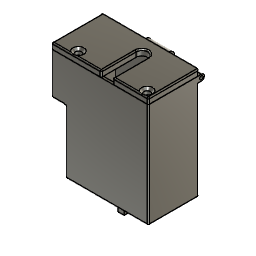
housing final project v8 (Autodesk Fusion 360 design; units mm, degrees)
Autodesk Fusion 360 part; units mm, degrees
note: some values were not read from the file. Set by a fixed rule: which face or edge a step refers to.
sketch "Sketch1" plane through (0, 0, 0) normal (0, 0, 1) x (1, 0, 0)
  line L0 (0, 0) -> (66.04, 0)
  line L1 (66.04, 0) -> (66.04, 38.1)
  line L2 (66.04, 38.1) -> (0, 38.1)
  line L3 (0, 38.1) -> (0, 0)
  line L4 (25.57, 28.525) -> (27.77, 28.525)
  line L5 (27.77, 28.525) -> (27.77, 19.825)
  line L6 (27.77, 19.825) -> (25.57, 19.825)
  line L7 (25.57, 19.825) -> (25.57, 28.525)
  line L8 (38.27, 27.675) -> (40.47, 27.675)
  line L9 (40.47, 27.675) -> (40.47, 20.675)
  line L10 (40.47, 20.675) -> (38.27, 20.675)
  line L11 (38.27, 20.675) -> (38.27, 27.675)
  line L12 (30.32, 12.275) -> (35.72, 12.275) construction
  line L13 (35.72, 12.275) -> (35.72, 9.575)
  line L14 (35.72, 9.575) -> (30.32, 9.575)
  line L15 (30.32, 9.575) -> (30.32, 12.275)
  line L16 (26.67, 28.525) -> (26.67, 19.825) construction
  line L17 (39.37, 27.675) -> (39.37, 20.675) construction
  arc A0 (35.72, 12.275) -> (30.32, 12.275) centre (33.02, 12.275) ccw
  line L18 (40.47, 24.175) -> (38.27, 24.175) construction
  line L19 (25.57, 24.175) -> (27.77, 24.175) construction
  dimension "d1" = 66.04
  dimension "d2" = 38.1
  dimension "d3" = 8.7
  dimension "d4" = 2.2
  dimension "d5" = 7
  dimension "d6" = 2.2
  dimension "d7" = 12.7
  dimension "d8" = 5.4
  dimension "d9" = 5.4
  dimension "d10" = 2.7
  dimension "d11" = 2.7
  dimension "d12" = 11.9
  dimension "d13" = 6.35
  dimension "d14" = 33.02
  dimension "d15" = 9.575
  constraint horizontal L0
  constraint vertical L1
  constraint horizontal L2
  constraint vertical L3
  constraint coincident L0.start L3.end
  constraint horizontal L4
  constraint vertical L5
  constraint horizontal L6
  constraint vertical L7
  constraint horizontal L8
  constraint vertical L9
  constraint horizontal L10
  constraint vertical L11
  constraint horizontal L12
  constraint vertical L13
  constraint horizontal L14
  constraint vertical L15
  constraint midpoint L4 L16.start
  constraint midpoint L6 L16.end
  constraint midpoint L8 L17.start
  constraint midpoint L10 L17.end
  constraint tangent L13 A0
  constraint midpoint L9 L18.start
  constraint midpoint L11 L18.end
  constraint midpoint L7 L19.start
  constraint midpoint L5 L19.end
  constraint collinear L18 L19
  measures "d1" distance of L1.end L2.end
  measures "d2" distance of L0.end L1.end
  measures "d3" distance of L4 L6
  measures "d4" distance of L4.start L4.end
  measures "d5" distance of L8.start L10.end
  measures "d6" distance of L8.start L8.end
  measures "d7" distance of L16 L17
  measures "d8" distance of L13.end L14.end
  measures "d9" diameter of A0
  measures "d10" distance of L14 A0.centre
  measures "d11" distance of L12.end L13.end
  measures "d12" distance of L12.end L18
  measures "d13" distance of L16 A0.centre
  measures "d14" distance of L1 A0.centre
  measures "d15" distance of L2 L4
extrude "Extrude1" add sketch "Sketch1" against normal blind 40.64 contours L0 L1 L2 L3 | L4 L5 L6 L7 | L8 L9 L10 L11 | L13 L14 L15 A0 makes body 1
extrude "Extrude2" cut sketch "Sketch1" against normal blind 15 contours L4 L5 L6 L7 | L8 L9 L10 L11 | L13 L14 L15 A0 bodies 1
extrude "Extrude3" add sketch "Sketch1" against normal blind 15 from surface at -40.64 contours L4 L5 L6 L7 | L8 L9 L10 L11 | L13 L14 L15 A0 bodies 1
sketch "Sketch3" plane through (25.57, 0, 0) normal (-1, 0, 0) x (0, -1, 0)
  line L0 (-19.825, -40.64) -> (-28.525, -40.64)
  circle A0 centre (-24.175, -50.64) radius 2
  line L1 (-24.175, -55.14) -> (-24.175, -40.64) construction
  line L2 (-28.525, -40.64) -> (-28.525, -55.64)
  line L3 (-28.525, -55.64) -> (-19.825, -55.64)
  line L4 (-19.825, -55.64) -> (-19.825, -40.64)
  dimension "d43" = 4
  constraint midpoint L0 L1.end
  constraint coincident A0.centre L1
  measures "d43" diameter of A0
sketch "Sketch2" plane through (66.04, 0, 0) normal (1, 0, 0) x (0, 1, 0)
  line L0 (35.1, -3) -> (3, -37.64) construction
  line L1 (35.1, -37.64) -> (3, -3) construction
  line L2 (25.55, -26.82) -> (12.55, -26.82)
  line L3 (12.55, -26.82) -> (12.55, -13.82)
  line L4 (12.55, -13.82) -> (25.55, -13.82)
  line L5 (25.55, -13.82) -> (25.55, -26.82)
  line L6 (25.55, -26.82) -> (12.55, -13.82) construction
  line L7 (12.55, -26.82) -> (25.55, -13.82) construction
  circle A0 centre (24.05, -15.32) radius 1.5
  line L8 (25.55, -20.32) -> (12.55, -20.32) construction
  line L9 (19.05, -13.82) -> (19.05, -26.82) construction
  circle A1 centre (24.05, -25.32) radius 1.5
  circle A2 centre (14.05, -15.32) radius 1.5
  circle A3 centre (14.05, -25.32) radius 1.5
  line L10 (38.1, 0) -> (0, 0)
  line L11 (0, 0) -> (0, -40.64)
  line L12 (0, -40.64) -> (38.1, -40.64)
  line L13 (38.1, -40.64) -> (38.1, 0)
  point P0 (19.05, -20.32)
  dimension "d27" = 13
  dimension "d28" = 13
  dimension "d29" = 3
  constraint horizontal L2
  constraint perpendicular L2 L3
  constraint parallel L2 L4
  constraint parallel L3 L5
  constraint coincident L6 P0
  constraint coincident L7 P0
  constraint tangent L5 A0
  constraint tangent L4 A0
  constraint midpoint L5 L8.start
  constraint midpoint L3 L8.end
  constraint midpoint L4 L9.start
  constraint midpoint L2 L9.end
  constraint symmetric A0 L8 A1
  constraint symmetric A0 L9 A2
  constraint symmetric L9 A1 A3
  constraint midpoint L1 P0
  measures "d27" distance of L2.start L2.end
  measures "d28" distance of L2.start L4.end
  measures "d29" diameter of A0
extrude "Extrude6" cut sketch "Sketch3" against normal up to surface (14.9 mm away) contours A0 bodies 1
extrude "Extrude5" add sketch "Sketch2" against normal blind 1 from surface at -66.04 contours L2 L3 L4 L5 A0 A1 A2 A3 | A1 | A3 | A0 | A2 bodies 1
extrude "Extrude4" add sketch "Sketch2" along normal blind 1 contours L2 L3 L4 L5 A0 A1 A2 A3 | A1 | A3 | A0 | A2 bodies 1
sketch "Sketch5" plane through (0, 0, -40.64) normal (0, 0, -1) x (1, 0, 0)
  line L0 (30.32, -12.275) -> (30.32, -9.575)
  line L1 (30.32, -9.575) -> (35.72, -9.575)
  line L2 (35.72, -9.575) -> (35.72, -12.275)
  arc A0 (30.32, -12.275) -> (35.72, -12.275) centre (33.02, -12.275) ccw
  line L3 (40.47, -27.675) -> (38.27, -27.675)
  line L4 (38.27, -27.675) -> (38.27, -20.675)
  line L5 (38.27, -20.675) -> (40.47, -20.675)
  line L6 (40.47, -20.675) -> (40.47, -27.675)
  line L7 (27.77, -28.525) -> (25.57, -28.525)
  line L8 (25.57, -28.525) -> (25.57, -19.825)
  line L9 (25.57, -19.825) -> (27.77, -19.825)
  line L10 (27.77, -19.825) -> (27.77, -28.525)
  line L11 (0, 0) -> (0, -38.1)
  line L12 (0, -38.1) -> (66.04, -38.1)
  line L13 (66.04, -38.1) -> (66.04, 0)
  line L14 (66.04, 0) -> (0, 0)
  line L15 (-0.5, -38.6) -> (66.54, -38.6)
  line L16 (66.54, -38.6) -> (66.54, 0.5)
  line L17 (66.54, 0.5) -> (-0.5, 0.5)
  line L18 (-0.5, 0.5) -> (-0.5, -38.6)
  line L19 (-2.5, 2.5) -> (-2.5, -40.6)
  line L20 (-2.5, -40.6) -> (68.54, -40.6)
  line L21 (68.54, -40.6) -> (68.54, 2.5)
  line L22 (68.54, 2.5) -> (-2.5, 2.5)
  dimension "d47" = 0.5
  dimension "d48" = 0.5
  dimension "d49" = 0.5
  dimension "d50" = 0.5
  dimension "d51" = 2
  constraint horizontal L15
  constraint vertical L16
  constraint horizontal L17
  constraint vertical L18
  measures "d47" distance of L13 L16
  measures "d48" distance of L11 L18
  measures "d49" distance of L12 L15
  measures "d50" distance of L14 L17
fillet "Fillet2" radius 1.5 4 edges at (26.67, 28.525, -55.64) (26.67, 19.825, -55.64) (39.37, 20.675, -55.64) (39.37, 27.675, -55.64) on bodies 1
fillet "Fillet3" radius 0.5 10 edges at (38.27, 20.675, -47.39) (38.27, 21.1143, -55.2007) (38.27, 24.175, -55.64) (38.27, 27.2357, -55.2007) (38.27, 27.675, -47.39) (40.47, 27.675, -47.39) (40.47, 27.2357, -55.2007) (40.47, 24.175, -55.64) (40.47, 21.1143, -55.2007) (40.47, 20.675, -47.39) on bodies 1
fillet "Fillet4" radius 0.5 10 edges at (27.77, 28.525, -47.39) (27.77, 28.0857, -55.2007) (27.77, 24.175, -55.64) (27.77, 20.2643, -55.2007) (27.77, 19.825, -47.39) (25.57, 19.825, -47.39) (25.57, 20.2643, -55.2007) (25.57, 24.175, -55.64) (25.57, 28.0857, -55.2007) (25.57, 28.525, -47.39) on bodies 1
fillet "Fillet5" radius 0.5 4 edges at (30.32, 10.925, -55.64) (33.02, 14.975, -55.64) (35.72, 10.925, -55.64) (33.02, 9.575, -55.64) on bodies 1
fillet "Fillet1" radius 3 12 edges at (0, 19.05, 0) (33.02, 38.1, 0) (66.04, 19.05, 0) (33.02, 0, 0) (0, 38.1, -20.32) (0, 0, -20.32) (0, 19.05, -40.64) (33.02, 0, -40.64) (66.04, 0, -20.32) (66.04, 19.05, -40.64) (66.04, 38.1, -20.32) (33.02, 38.1, -40.64) on bodies 1
chamfer "Chamfer1" distance 0.5 angle 45 12 edges at (26.67, 28.525, 0) (25.57, 24.175, 0) (27.77, 24.175, 0) (26.67, 19.825, 0) (39.37, 27.675, 0) (38.27, 24.175, 0) (40.47, 24.175, 0) (39.37, 20.675, 0) (33.02, 14.975, 0) (35.72, 10.925, 0) (30.32, 10.925, 0) (33.02, 9.575, 0) on bodies 1
extrude "Extrude7" add sketch "Sketch5" against normal blind 90 separate body contours L19 L20 L21 L22 makes body 2
sketch "Sketch6" plane through (-2.5, 0, 0) normal (-1, 0, 0) x (0, -1, 0)
  line L0 (-40.6, -40.64) -> (2.5, -40.64)
  line L1 (2.5, -40.64) -> (2.5, 49.36)
  line L2 (2.5, 49.36) -> (-40.6, 49.36)
  line L3 (-40.6, 49.36) -> (-40.6, -40.64)
  line L4 (-40.6, 0.36) -> (2.5, 0.36)
  line L5 (-40.6, 2.36) -> (2.5, 2.36)
  line L6 (-7.5, 2.36) -> (-7.5, 0.36)
  line L7 (-30.6, 2.36) -> (-30.6, 0.36)
  dimension "d54" = 41
  dimension "d55" = 2
  dimension "d56" = 10
  dimension "d57" = 10
  constraint coincident L3 L4.start
  constraint coincident L1 L4.end
  constraint perpendicular L1 L4
  constraint coincident L3 L5.start
  constraint coincident L1 L5.end
  constraint perpendicular L1 L5
  constraint coincident L5 L6.start
  constraint coincident L4 L6.end
  constraint perpendicular L4 L6
  constraint coincident L5 L7.start
  constraint coincident L4 L7.end
  constraint perpendicular L4 L7
  measures "d54" distance of L0 L4
  measures "d55" distance of L4 L5
  measures "d56" distance of L1 L6
  measures "d57" distance of L3 L7
extrude "Extrude8" add sketch "Sketch6" against normal blind 10 from surface at -2 contours L3 L4 L5 L7 | L1 L4 L5 L6 | L4 L5 L6 L7 bodies 2
extrude "Extrude9" add sketch "Sketch6" along normal blind 10 from surface at -69.04 contours L3 L4 L5 L7 | L1 L4 L5 L6 | L4 L5 L6 L7 bodies 2
chamfer "Chamfer2" distance 10 angle 45 2 edges at (-0.5, 19.05, 2.36) (66.54, 19.05, 2.36) on bodies 2
sketch "Sketch8" plane through (68.54, 0, 0) normal (1, 0, 0) x (0, 1, 0)
  line L0 (-2.5, -40.64) -> (40.6, -40.64)
  line L1 (40.6, -40.64) -> (40.6, 49.36)
  line L2 (40.6, 49.36) -> (-2.5, 49.36)
  line L3 (-2.5, 49.36) -> (-2.5, -40.64)
  line L4 (40.6, 49.36) -> (43.1, 49.36)
  line L5 (43.1, 49.36) -> (43.1, 44.36)
  line L6 (43.1, 44.36) -> (40.6, 44.36)
  line L7 (40.6, 44.36) -> (40.6, 49.36)
  circle A0 centre (43.1, 46.86) radius 2.5
  circle A1 centre (43.1, 46.86) radius 1.5
  line L8 (-2.5, 49.36) -> (7.5, 49.36)
  line L9 (7.5, 49.36) -> (7.5, 39.36)
  line L10 (7.5, 39.36) -> (-2.5, 39.36)
  line L11 (-2.5, 39.36) -> (-2.5, 49.36)
  line L12 (-0.5, 39.36) -> (-0.5, 49.36)
  dimension "d65" = 5
  dimension "d66" = 2.5
  dimension "d67" = 5
  dimension "d73" = 3
  dimension "d76" = 10
  dimension "d77" = 10
  dimension "d78" = 2
  constraint horizontal L4
  constraint vertical L5
  constraint horizontal L6
  constraint vertical L7
  constraint coincident L1.end L2.start
  constraint midpoint L5 A0.centre
  constraint concentric A0 A1
  constraint horizontal L8
  constraint vertical L9
  constraint horizontal L10
  constraint vertical L11
  constraint coincident L2.end L3.start
  constraint coincident L10 L12.start
  constraint coincident L8 L12.end
  constraint perpendicular L8 L12
  measures "d65" distance of L4.end L5.end
  measures "d66" distance of L1.end L4.end
  measures "d67" diameter of A0
  measures "d73" diameter of A1
  measures "d76" distance of L9.end L10.end
  measures "d77" distance of L8.end L9.end
  measures "d78" distance of L11 L12
extrude "Extrude10" add sketch "Sketch8" against normal blind 25 contours L1 L6 L7 A0 | L1 L4 L7 A0 | L5 A0 A1 | L5 A0 A1 | L5 A1 | L5 A1 bodies 2
extrude "Extrude11" add sketch "Sketch8" along normal blind 25 from surface at -71.04 contours L1 L6 L7 A0 | L1 L4 L7 A0 | L5 A0 A1 | L5 A0 A1 | L5 A1 | L5 A1 bodies 2
extrude "Extrude12" cut sketch "Sketch8" against normal up to surface (71.04 mm away) contours L5 A1 | L5 A1 bodies 2
extrude "Extrude13" add sketch "Sketch8" against normal blind 10 from surface at -2 contours L2 L8 L9 L10 L12 bodies 2
extrude "Extrude14" add sketch "Sketch8" along normal blind 10 from surface at -69.04 contours L2 L8 L9 L10 L12 bodies 2
sketch "Sketch10" plane through (-2.5, 0, 0) normal (-1, 0, 0) x (0, -1, 0)
  circle A0 centre (-43.1, 46.86) radius 1.5
  line L0 (-40.6, -40.64) -> (2.5, -40.64)
  line L1 (2.5, -40.64) -> (2.5, 49.36)
  line L2 (2.5, 49.36) -> (-43.1, 49.36)
  arc A1 (-43.1, 49.36) -> (-43.1, 44.36) centre (-43.1, 46.86) ccw
  line L3 (-43.1, 44.36) -> (-40.6, 44.36)
  line L4 (-40.6, 44.36) -> (-40.6, -40.64)
  line L5 (2.5, 54.46) -> (-40.6, 54.46)
  line L6 (-40.6, 54.46) -> (-40.6, 49.46)
  line L7 (-40.6, 49.46) -> (2.5, 49.46)
  line L8 (2.5, 49.46) -> (2.5, 54.46)
  line L9 (2.5, 39.36) -> (2.5, 49.36)
  circle A2 centre (-43.1, 46.86) radius 2.5
  dimension "d88" = 0.1
  dimension "d89" = 5
  constraint horizontal L5
  constraint vertical L6
  constraint horizontal L7
  constraint vertical L8
  constraint collinear L8 L9
  constraint collinear L4 L6
  measures "d88" distance of L2 L7
  measures "d89" distance of L5.start L7.end
extrude "Extrude16" add sketch "Sketch10" against normal up to surface (71.04 mm away) separate body contours L5 L6 L7 L8 makes body 3
sketch "Sketch12" plane through (0, 40.6, 0) normal (0, 1, 0) x (-1, 0, 0)
  line L0 (-68.54, 54.46) -> (-68.54, 49.46)
  line L1 (-68.54, 49.46) -> (2.5, 49.46)
  line L2 (2.5, 49.46) -> (2.5, 54.46)
  line L3 (2.5, 54.46) -> (-68.54, 54.46)
  line L4 (-33.02, 54.46) -> (-33.02, 49.46) construction
  line L5 (-23.02, 54.46) -> (-23.02, 49.46)
  line L6 (-43.02, 54.46) -> (-43.02, 49.46)
  dimension "d92" = 10
  constraint midpoint L3 L4.start
  constraint midpoint L1 L4.end
  constraint coincident L3 L5.start
  constraint coincident L1 L5.end
  constraint perpendicular L1 L5
  constraint symmetric L4 L5.start L6.start
  constraint symmetric L4 L5.end L6.end
  measures "d92" distance of L4 L5
extrude "Extrude17" add sketch "Sketch12" along normal blind 5 contours L1 L3 L5 L6 bodies 3
sketch "Sketch14" plane through (23.02, 0, 0) normal (-1, 0, 0) x (0, -1, 0)
  line L0 (-40.6, 49.46) -> (-40.6, 54.46)
  line L1 (-40.6, 54.46) -> (-45.6, 54.46)
  line L2 (-45.6, 54.46) -> (-45.6, 49.46)
  line L3 (-45.6, 49.46) -> (-40.6, 49.46)
  line L4 (-45.6, 49.46) -> (-40.6, 49.46)
  line L5 (-40.6, 49.46) -> (-40.6, 44.36)
  line L6 (-40.6, 44.36) -> (-45.6, 44.36)
  line L7 (-45.6, 44.36) -> (-45.6, 49.46)
  line L8 (-40.6, 49.36) -> (-45.6, 49.36)
  line L9 (-45.6, 49.36) -> (-40.6, 44.36) construction
  line L10 (-40.6, 49.36) -> (-45.6, 44.36) construction
  circle A0 centre (-43.1, 46.86) radius 2.5
  circle A1 centre (-43.1, 46.86) radius 1.5
  dimension "d96" = 5.1
  dimension "d97" = 5
  dimension "d98" = 0.1
  dimension "d99" = 5
  dimension "d100" = 3
  constraint horizontal L4
  constraint vertical L5
  constraint horizontal L6
  constraint vertical L7
  constraint coincident L2.end L3.start
  constraint coincident L5 L8.start
  constraint coincident L7 L8.end
  constraint perpendicular L7 L8
  constraint midpoint L10 A0.centre
  constraint concentric A0 A1
  measures "d96" distance of L2.end L6.end
  measures "d97" distance of L5.end L6.end
  measures "d98" distance of L4 L8
  measures "d99" diameter of A0
  measures "d100" diameter of A1
sketch "Sketch9" plane through (0, 0, 49.36) normal (0, 0, 1) x (-1, 0, 0)
  line L0 (0.5, -7.5) -> (0.5, -38.6)
  line L1 (0.5, -38.6) -> (-66.54, -38.6)
  line L2 (-66.54, -38.6) -> (-66.54, -7.5)
  line L3 (-66.54, -7.5) -> (-56.54, -7.5)
  line L4 (-56.54, -7.5) -> (-56.54, 0.5)
  line L5 (-56.54, 0.5) -> (-9.5, 0.5)
  line L6 (-9.5, 0.5) -> (-9.5, -7.5)
  line L7 (-9.5, -7.5) -> (0.5, -7.5)
  line L8 (2.5, 2.5) -> (-68.54, 2.5)
  line L9 (-68.54, 2.5) -> (-68.54, -43.1)
  line L10 (-68.54, -43.1) -> (-43.54, -43.1)
  line L11 (-43.54, -43.1) -> (-43.54, -40.6)
  line L12 (-43.54, -40.6) -> (-22.5, -40.6)
  line L13 (-22.5, -40.6) -> (-22.5, -43.1)
  line L14 (-22.5, -43.1) -> (2.5, -43.1)
  line L15 (2.5, -43.1) -> (2.5, 2.5)
  line L16 (-9.5, -7.5) -> (2.5, 2.5) construction
  line L17 (0.5, -7.5) -> (2.5, -7.5) construction
  line L18 (-9.5, 0.5) -> (-9.5, 2.5) construction
  line L19 (-9.5, 2.5) -> (2.5, -7.5) construction
  circle A0 centre (-3.5, -2.5) radius 2.7
  line L20 (-33.02, 2.5) -> (-33.02, 0.5) construction
  circle A1 centre (-62.54, -2.5) radius 2.7
  dimension "d85" = 5.4
  constraint coincident L6.end L7.start
  constraint coincident L8.start L15.end
  constraint coincident L0.start L7.end
  constraint coincident L15 L17.end
  constraint perpendicular L15 L17
  constraint coincident L5.end L6.start
  constraint coincident L8 L18.end
  constraint perpendicular L8 L18
  constraint midpoint L16 A0.centre
  constraint midpoint L8 L20.start
  constraint midpoint L5 L20.end
  constraint symmetric A0 L20 A1
  measures "d85" diameter of A0
extrude "Extrude15" cut sketch "Sketch9" against normal up to surface (10 mm away) contours A0 | A1 bodies 2
extrude "Extrude18" add sketch "Sketch14" against normal up to surface (20 mm away) contours L3 L4 L5 L7 L8 | L5 L8 A0 | L7 L8 A0 | A0 bodies 3
extrude "Extrude19" cut sketch "Sketch9" along normal up to surface (5.1 mm away) contours A0 | A1 bodies 3
sketch "Sketch15" plane through (0, 0, 54.46) normal (0, 0, 1) x (-1, 0, 0)
  circle A0 centre (-3.5, -2.5) radius 2.7
  circle A1 centre (-62.54, -2.5) radius 2.7
  line L0 (-68.54, 2.5) -> (-68.54, -40.6)
  line L1 (-68.54, -40.6) -> (-43.02, -40.6)
  line L2 (-43.02, -40.6) -> (-43.02, -45.6)
  line L3 (-43.02, -45.6) -> (-23.02, -45.6)
  line L4 (-23.02, -45.6) -> (-23.02, -40.6)
  line L5 (-23.02, -40.6) -> (2.5, -40.6)
  line L6 (2.5, -40.6) -> (2.5, 2.5)
  line L7 (2.5, 2.5) -> (-68.54, 2.5)
  line L8 (-33.02, -45.6) -> (-33.02, 2.5) construction
  line L9 (-38.02, -27.5) -> (-28.02, -27.5)
  line L10 (-28.02, -27.5) -> (-28.02, 2.5)
  line L11 (-28.02, 2.5) -> (-38.02, 2.5)
  line L12 (-38.02, 2.5) -> (-38.02, -27.5)
  line L13 (-38.02, -27.5) -> (-28.02, 2.5) construction
  line L14 (-28.02, -27.5) -> (-38.02, 2.5) construction
  circle A2 centre (-33.02, -27.5) radius 5
  point P0 (-33.02, -12.5)
  dimension "d107" = 30
  dimension "d108" = 10
  dimension "d109" = 10
  constraint midpoint L3 L8.start
  constraint midpoint L7 L8.end
  constraint horizontal L9
  constraint perpendicular L9 L10
  constraint parallel L9 L11
  constraint parallel L10 L12
  constraint coincident L13 P0
  constraint coincident L14 P0
  constraint coincident L8 P0
  constraint collinear L7 L11
  constraint midpoint L9 A2.centre
  measures "d107" distance of L9.start L11.end
  measures "d108" distance of L9.start L9.end
  measures "d109" diameter of A2
extrude "Extrude20" cut sketch "Sketch15" against normal up to surface (5 mm away) contours L7 L10 L11 L12 A2 | L9 A2 | L9 A2 bodies 3
fillet "Fillet6" radius 5 1 edges at (33.02, 45.6, 54.46) on bodies 3
chamfer "Chamfer3" distance 2 angle 45 2 edges at (6.0173, 1.5236, 54.46) (65.0573, 1.5236, 54.46) on bodies 3
sketch "Sketch19" plane through (-2.5, 0, 0) normal (-1, 0, 0) x (0, -1, 0)
  line L0 (-40.6, -40.64) -> (2.5, -40.64)
  line L1 (2.5, 49.36) -> (-43.1, 49.36)
  arc A0 (-43.1, 49.36) -> (-43.1, 44.36) centre (-43.1, 46.86) ccw
  line L2 (-43.1, 44.36) -> (-40.6, 44.36)
  circle A1 centre (-43.1, 46.86) radius 1.5
  line L3 (-2.3867, 49.36) -> (-2.3867, 15.36)
  line L4 (-2.3867, 15.36) -> (-36.3867, 15.36)
  line L5 (-36.3867, 15.36) -> (-36.3867, 49.36)
  line L6 (-19.05, -40.64) -> (-19.05, 49.36) construction
  line L7 (2.5, -40.64) -> (2.5, 49.36)
  line L8 (-40.6, 44.36) -> (-40.6, -40.64)
  line L9 (-40.6, 13.36) -> (2.5, 13.36)
  line L10 (-40.6, 44.36) -> (-40.6, 49.36)
  dimension "d140" = 34
  dimension "d141" = 34
  dimension "d156" = 2
  constraint vertical L3
  constraint horizontal L4
  constraint vertical L5
  constraint midpoint L0 L6.start
  constraint coincident L1 L6.end
  constraint perpendicular L1 L6
  constraint coincident L1 L3.start
  constraint coincident L8 L9.start
  constraint coincident L7 L9.end
  constraint perpendicular L7 L9
  constraint coincident L2.end L8.start
  constraint coincident L1 L10.end
  constraint perpendicular L1 L10
  measures "d140" distance of L5.end L3.start
  measures "d141" distance of L5.end L4.end
  measures "d156" distance of L4 L9
extrude "Extrude22" add sketch "Sketch19" along normal blind 10 contours L1 L3 L4 L5 L7 L8 L9 L10 bodies 2
extrude "Extrude23" add sketch "Sketch19" along normal blind 2 from surface at 10 contours L1 L3 L4 L5 L7 L8 L9 L10 | L1 L3 L4 L5 bodies 2
extrude "Extrude24" add 1 faces at (-2.5, 26.2333, 51.1267) along direction (-1, 0, 0) blind 12 on bodies 3 bodies 3
fillet "Fillet8" radius 1 3 edges at (68.54, 40.6, 1.86) (-2.5, 40.6, -13.64) (-2.5, 40.6, 46.86) on bodies 2
fillet "Fillet8" radius 1 11 edges at (-14.5, -2.5, 31.36) (-8.5, -2.5, 13.36) (-14.5, 19.05, 13.36) (-14.5, 40.6, 31.36) (-8.5, 40.6, 13.36) (-2.5, 19.05, 13.36) (-2.5, -2.5, -13.64) (-2.5, 19.05, -40.64) (33.02, -2.5, -40.64) (33.02, 40.6, -40.64) (68.54, 19.05, -40.64) on bodies 2
fillet "Fillet8" radius 1 1 edges at (68.54, -2.5, 4.36) on bodies 2
fillet "Fillet9" radius 1 8 edges at (68.54, 40.6, 51.96) (68.54, 19.05, 54.46) (68.54, -2.5, 51.96) (53.28, -2.5, 54.46) (28.02, 12.5, 54.46) (33.02, 32.5, 54.46) (38.02, 12.5, 54.46) (38.02, -2.5, 51.96) on bodies 3
fillet "Fillet9" radius 1 5 edges at (6.76, -2.5, 54.46) (-14.5, 19.05, 54.46) (-14.5, 40.6, 51.96) (-14.5, -2.5, 51.96) (28.02, -2.5, 51.96) on bodies 3
sketch "Sketch21" plane through (0, 40.6, 0) normal (0, 1, 0) x (-1, 0, 0)
  line L0 (3.5, 49.36) -> (3.5, 44.36)
  line L1 (3.5, 44.36) -> (-22.5, 44.36)
  line L2 (-22.5, 44.36) -> (-22.5, 49.36)
  line L3 (-22.5, 49.36) -> (-43.54, 49.36)
  line L4 (-43.54, 49.36) -> (-43.54, 44.36)
  line L5 (-43.54, 44.36) -> (-67.54, 44.36)
  line L6 (-67.54, 44.36) -> (-67.54, -39.64)
  line L7 (-67.54, -39.64) -> (1.5, -39.64)
  line L8 (1.5, -39.64) -> (1.5, 12.36)
  arc A0 (3.5, 14.36) -> (1.5, 12.36) centre (3.5, 12.36) ccw
  line L9 (3.5, 14.36) -> (13.5, 14.36)
  line L10 (13.5, 14.36) -> (13.5, 49.36)
  line L11 (13.5, 49.36) -> (3.5, 49.36)
  line L12 (-58.02, 5.36) -> (-8.02, 5.36)
  line L13 (-8.02, 5.36) -> (-8.02, -19.64)
  line L14 (-8.02, -19.64) -> (-58.02, -19.64)
  line L15 (-58.02, -19.64) -> (-58.02, 5.36)
  line L16 (-33.02, -39.64) -> (-33.02, 50.36) construction
  line L17 (-49.0719, 15.4014) -> (-17.0719, 15.4014) construction
  line L18 (-17.0719, 15.4014) -> (-17.0719, 29.4014) construction
  line L19 (-17.0719, 29.4014) -> (-49.0719, 29.4014) construction
  line L20 (-49.0719, 29.4014) -> (-49.0719, 15.4014) construction
  dimension "d163" = 25
  dimension "d164" = 50
  dimension "d165" = 20
  dimension "d166" = 8
  text T0 "Lacime" font "Arial" height 8 italic align centre top in box 32 x 14 at (-49.0719, 15.4014) x (1, 0) y (0, 1) spacing 1 kerned
  constraint horizontal L12
  constraint vertical L13
  constraint horizontal L14
  constraint vertical L15
  constraint midpoint L7 L16.start
  constraint perpendicular L7 L16
  constraint midpoint L12 L16
  measures "d163" distance of L12.end L13.end
  measures "d164" distance of L12.start L12.end
  measures "d165" distance of L7 L14
extrude "Extrude25" cut sketch "Sketch21" sketch "Sketch21" against normal blind 0.5 contours L12 L13 L14 L15 of sketch 2 text T0 bodies 2
chamfer "Chamfer5" distance 0.5 angle 45 4 edges at (33.02, 40.6, 5.36) (58.02, 40.6, -7.14) (33.02, 40.6, -19.64) (8.02, 40.6, -7.14) on bodies 2
copy_body "Body->Comp4" bodies 3 removing the originals makes body 4 in component "Component"
copy_body "Body->Comp5" bodies 2 removing the originals makes body 5 in component "Component'"
copy_body "Body->Comp6" bodies 1 removing the originals makes body 6 in component "Component''"
component "Component" placed x (1, 0, 0) y (0, 1, 0) z (0, 0, 1) at (0, 0, 0)
component "Component'" placed x (1, 0, 0) y (0, 1, 0) z (0, 0, 1) at (0, 0, 0)
component "Component''" placed x (1, 0, 0) y (0, 1, 0) z (0, 0, 1) at (0, 0, 0)
equation "d10 = ( 5.4 / 2 ) * 1 mm"
equation "d11 = ( 5.4 / 2 ) * 1 mm"
equation "d13 = ( 12.7 / 2 ) * 1 mm"
equation "d14 = ( 66.04 / 2 ) * 1 mm"
